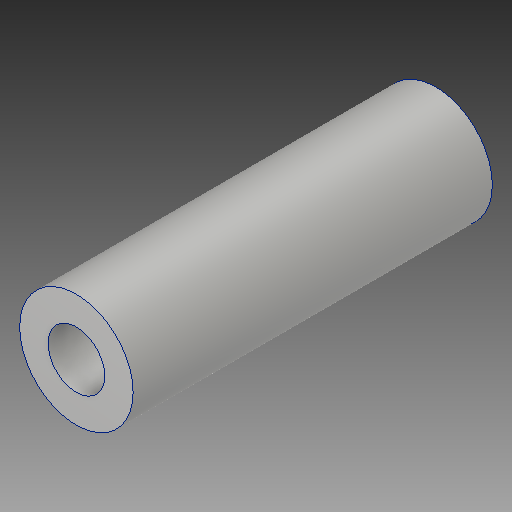
# Autodesk Inventor part: スペーサーm3,19
Saved by Autodesk Inventor 2017 (Build 210142000, 142)
## iProperties
Part Number: スペーサーm3,19
Material: アルミニウム 6061
Document SubType Name: Modeling
Designer: 雪村
Density: 2.7 g/cm^3
Appearance: アルミニウム - フラット
Mass: 1.08785 g
Surface Area: 5.79624 cm^2
Volume: 0.402909 cm^3
Author: 雪村
Autodesk Inventor part; units mm, degrees
ref_plane "YZ Plane" through (0, 0, 0) normal (1, 0, 0) x (0, 1, 0)
ref_plane "XZ Plane" through (0, 0, 0) normal (0, 1, 0) x (-1, 0, 0)
ref_plane "XY Plane" through (0, 0, 0) normal (0, 0, 1) x (1, 0, 0)
sketch "スケッチ1" plane through (0, 0, 0) normal (0, 0, 1) x (1, 0, 0)
  circle A0 centre (0, 0) radius 3
  circle A1 centre (0, 0) radius 1.5
  dimension "d0" = 6
  dimension "d1" = 3
  constraints: 2 centre point, 2 coincident
  measures "d0" diameter of A0
  measures "d1" diameter of A1
extrude "押し出し1" add sketch "スケッチ1" along normal blind 19
